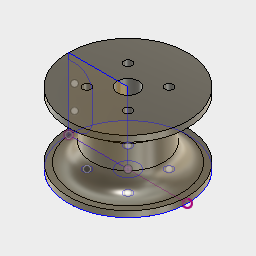
spool v2 (Autodesk Fusion 360 design; units mm, degrees)
Autodesk Fusion 360 part; units mm, degrees
sketch "Sketch1" plane through (0, 0, 0) normal (0, 0, 1) x (1, 0, 0)
  circle A0 centre (-6.915, -6.915) radius 1.4
  circle A1 centre (-6.915, 6.915) radius 1.4
  circle A2 centre (6.915, 6.915) radius 1.4
  circle A3 centre (6.915, -6.915) radius 1.4
  circle A4 centre (0, 0) radius 20
  circle A5 centre (0, 0) radius 3.5
  dimension "d3" = 2.8
  dimension "d4" = 2.8
  dimension "d5" = 2.8
  dimension "d6" = 2.8
  dimension "d22" = 7
  constraint coincident A4
  constraint concentric A4 A5
  measures "d3" diameter of A0
  measures "d4" diameter of A1
  measures "d5" diameter of A3
  measures "d6" diameter of A2
  measures "d22" diameter of A5
sketch "Sketch7" plane through (0, 0, 0) normal (0, 1, 0) x (1, 0, 0)
  line L0 (0, 0) -> (-20, 0)
  line L1 (-20, 0) -> (-20, -24)
  line L2 (-20, -24) -> (0, -24)
  line L3 (0, -24) -> (0, 0)
  line L4 (-20, 0) -> (20, 0)
  line L5 (-20, -24) -> (-20, -22)
  line L6 (-20, 0) -> (-20, -2)
  line L7 (-20, -22) -> (-18, -22)
  line L8 (-20, -2) -> (-18, -2)
  line L9 (-12, -16) -> (-12, -8)
  arc A0 (-12, -8) -> (-18, -2) centre (-18, -8) ccw
  arc A1 (-18, -22) -> (-12, -16) centre (-18, -16) ccw
  dimension "d15" = 24
  dimension "d16" = 2
  dimension "d17" = 2
  dimension "d20" = 6
  dimension "d21" = 6
  constraint perpendicular L0 L1
  constraint parallel L0 L2
  constraint parallel L1 L3
  constraint parallel L0 L4
  constraint perpendicular L5 L7
  constraint tangent L8 A0
  constraint tangent L9 A0
  constraint tangent L7 A1
  constraint tangent L9 A1
  measures "d20" radius of A0
  measures "d21" radius of A1
revolve "Revolve1" add sketch "Sketch7" angle 360 about axis through (0, 0, 24) along (0, 0, -1) contours L0 L1 L2 L3 L4 L5 L6 L7 L8 L9 A0 A1
extrude "Extrude2" cut sketch "Sketch1" along normal up to surface (24 mm away) contours A5
extrude "Extrude3" cut sketch "Sketch1" along normal up to surface (24 mm away) contours A2
extrude "Extrude4" cut sketch "Sketch1" along normal up to surface (24 mm away) contours A3
extrude "Extrude5" cut sketch "Sketch1" along normal up to surface (24 mm away) contours A0
extrude "Extrude6" cut sketch "Sketch1" along normal up to surface (24 mm away) contours A1
